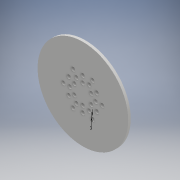
# Autodesk Inventor part: bottom-bearing-holder
Saved by Autodesk Inventor 2018 (Build 220112000, 112)
## iProperties
Created: 2024-05-26
Part Number: bottom-bearing-holder
Material: Generic
Document SubType Name: Modeling
Designer: neo
Density: 1 g/cm^3
Appearance: Default
Author: neo
Autodesk Inventor part; units mm, degrees
ref_plane "YZ Plane" through (0, 0, 0) normal (1, 0, 0) x (0, 1, 0)
ref_plane "XZ Plane" through (0, 0, 0) normal (0, 1, 0) x (-1, 0, 0)
ref_plane "XY Plane" through (0, 0, 0) normal (0, 0, 1) x (1, 0, 0)
sketch "Sketch1" plane through (0, 0, 0) normal (0, 0, 1) x (1, 0, 0)
  line L0 (0, 30.0543) -> (0, -31.5761)
  line L1 (40, 7.4457) -> (50, 7.4457)
  line L2 (50, 7.4457) -> (50, -2.5543)
  line L3 (50, -2.5543) -> (40, -2.5543)
  line L4 (40, -2.5543) -> (40, 7.4457)
  point P0 (0, 0)
  dimension "d0" = 10
  dimension "d1" = 10
  dimension "d2" = 80
  constraints: 10 end point, 2 parallel, 1 horizontal, 1 perpendicular, 1 point on line, 1 vertical
  measures "d0" distance of L1.start L1.end
  measures "d1" distance of L1.end L2.end
  measures "d2" diameter of L4 L0
revolve "Revolution1" add sketch "Sketch1" angle 360 about axis through (0, 30.0543, 0) along (0, -1, 0)
sketch "Sketch3" plane through (0, 7.4457, 0) normal (0, 1, 0) x (1, 0, 0)
  circle A0 centre (0, 0) radius 40 projected
  circle A1 centre (0, 0) radius 43
  point P0 (0, 0)
  dimension "d6" = 3
  constraints: 1 centre point, 1 coincident
  measures "d6" radial gap between concentric circles of A0 A1
extrude "Extrusion1" add sketch "Sketch3" along normal blind 4 contours A0 | A1
extrude "Extrusion2" add sketch "Sketch3" against normal blind 4 contours A0
sketch "Sketch4" plane through (0, -2.5543, 0) normal (0, -1, 0) x (1, 0, 0)
  circle A0 centre (0, 0) radius 40 projected
  circle A1 centre (0, 0) radius 43 projected
  point P0 (0, 0)
extrude "Extrusion3" add sketch "Sketch4" against normal blind 4 contours A0
extrude "Extrusion4" add sketch "Sketch4" along normal blind 4 contours A0 | A1
sketch "Sketch5" plane through (0, -6.5543, 0) normal (0, -1, 0) x (1, 0, 0)
  circle A0 centre (0, 0) radius 70
  dimension "d16" = 140
  constraints: 1 centre point, 1 coincident
  measures "d16" diameter of A0
extrude "Extrusion5" add sketch "Sketch5" along normal blind 4
sketch "Sketch6" plane through (0, 11.4457, 0) normal (0, 1, 0) x (1, 0, 0)
  circle A0 centre (0, 0) radius 30
  circle A1 centre (-30, 0) radius 1.5
  line L0 (0, 0) -> (-60.6002, 0)
  line L1 (0, 0) -> (-52.4813, -30.3001)
  line L2 (0, 0) -> (-30.3001, -52.4813)
  line L3 (0, 0) -> (0, -60.6002)
  line L4 (0, 0) -> (30.3001, -52.4813)
  line L5 (0, 0) -> (52.4813, -30.3001)
  line L6 (0, 0) -> (60.6002, 0)
  line L7 (0, 0) -> (52.4813, 30.3001)
  line L8 (0, 0) -> (30.3001, 52.4813)
  line L9 (0, 0) -> (0, 60.6002)
  line L10 (0, 0) -> (-30.3001, 52.4813)
  line L11 (0, 0) -> (-52.4813, 30.3001)
  circle A2 centre (0, 0) radius 20
  circle A3 centre (0, 0) radius 25
  circle A4 centre (0, 0) radius 15
  circle A5 centre (-21.6506, 12.5) radius 1.5
  circle A6 centre (-20, 0) radius 1.5
  circle A7 centre (-12.9904, 7.5) radius 1.5
  circle A8 centre (-15, -25.9808) radius 1.5
  circle A9 centre (-10, -17.3205) radius 1.5
  circle A10 centre (-21.6506, -12.5) radius 1.5
  circle A11 centre (-12.9904, -7.5) radius 1.5
  circle A12 centre (15, -25.9808) radius 1.5
  circle A13 centre (10, -17.3205) radius 1.5
  circle A14 centre (0, -25) radius 1.5
  circle A15 centre (0, -15) radius 1.5
  circle A16 centre (30, 0) radius 1.5
  circle A17 centre (20, 0) radius 1.5
  circle A18 centre (21.6506, -12.5) radius 1.5
  circle A19 centre (12.9904, -7.5) radius 1.5
  circle A20 centre (15, 25.9808) radius 1.5
  circle A21 centre (10, 17.3205) radius 1.5
  circle A22 centre (21.6506, 12.5) radius 1.5
  circle A23 centre (12.9904, 7.5) radius 1.5
  circle A24 centre (-15, 25.9808) radius 1.5
  circle A25 centre (-10, 17.3205) radius 1.5
  circle A26 centre (0, 25) radius 1.5
  circle A27 centre (0, 15) radius 1.5
  dimension "d19" = 60
  dimension "d25" = 40
  dimension "d26" = 50
  dimension "d27" = 30
  dimension "d20" = 3
  dimension "d23" = 360
  dimension "d28" = 3
  dimension "d29" = 3
  dimension "d30" = 3
  dimension "d33" = 360
  constraints: 24 centre point, 24 end point, 5 point on line, 3 coincident, 2 horizontal alignment, 1 horizontal, 96 other
  measures "d20" diameter of A1
  measures "d28" diameter of A5
  measures "d29" diameter of A6
  measures "d30" diameter of A7
hole "Hole1" at (-15, 11.4457, 25.9808) at (-30, 11.4457, 0) at (-15, 11.4457, -25.9808) at (15, 11.4457, -25.9808) at (30, 11.4457, 0) at (15, 11.4457, 25.9808) at (0, 11.4457, 25) at (-21.6506, 11.4457, 12.5) at (-21.6506, 11.4457, -12.5) at (-10, 11.4457, -17.3205) at (10, 11.4457, -17.3205) at (20, 11.4457, 0) at (21.6506, 11.4457, 12.5) at (21.6506, 11.4457, -12.5) at (12.9904, 11.4457, -7.5) at (12.9904, 11.4457, 7.5) at (10, 11.4457, 17.3205) at (0, 11.4457, 15) at (-10, 11.4457, 17.3205) at (-12.9904, 11.4457, 7.5) at (-20, 11.4457, 0) at (-12.9904, 11.4457, -7.5) at (0, 11.4457, -15) at (0, 11.4457, -25) direction (0, -1, 0) diameter 3 end through all counterbore diameter 6 counterbore depth 4
sketch "Sketch7" plane through (0, -10.5543, 0) normal (0, -1, 0) x (1, 0, 0)
  circle A0 centre (0, -15) radius 1.5 projected
  circle A1 centre (-20, 0) radius 1.5 projected
  circle A2 centre (-10, 17.3205) radius 1.5 projected
  circle A3 centre (10, 17.3205) radius 1.5 projected
  circle A4 centre (12.9904, -7.5) radius 1.5 projected
  circle A5 centre (21.6506, 12.5) radius 1.5 projected
  circle A6 centre (10, -17.3205) radius 1.5 projected
  circle A7 centre (-21.6506, -12.5) radius 1.5 projected
  circle A8 centre (0, 25) radius 1.5 projected
  circle A9 centre (30, 0) radius 1.5 projected
  circle A10 centre (-15, -25.9808) radius 1.5 projected
  circle A11 centre (-15, 25.9808) radius 1.5 projected
  circle A12 centre (-30, 0) radius 1.5 projected
  circle A13 centre (15, -25.9808) radius 1.5 projected
  circle A14 centre (15, 25.9808) radius 1.5 projected
  circle A15 centre (-21.6506, 12.5) radius 1.5 projected
  circle A16 centre (-10, -17.3205) radius 1.5 projected
  circle A17 centre (20, 0) radius 1.5 projected
  circle A18 centre (21.6506, -12.5) radius 1.5 projected
  circle A19 centre (12.9904, 7.5) radius 1.5 projected
  circle A20 centre (0, 15) radius 1.5 projected
  circle A21 centre (-12.9904, 7.5) radius 1.5 projected
  circle A22 centre (-12.9904, -7.5) radius 1.5 projected
  circle A23 centre (0, -25) radius 1.5 projected
  circle A24 centre (0, 0) radius 70 projected
  point P0 (0, 0)
hole "Hole2" at (30, -10.5543, 0) at (21.6506, -10.5543, -12.5) at (20, -10.5543, 0) at (21.6506, -10.5543, 12.5) at (15, -10.5543, 25.9808) at (12.9904, -10.5543, 7.5) at (12.9904, -10.5543, -7.5) at (15, -10.5543, -25.9808) at (10, -10.5543, -17.3205) at (0, -10.5543, -15) at (0, -10.5543, -25) at (0, -10.5543, 15) at (0, -10.5543, 25) at (10, -10.5543, 17.3205) at (-10, -10.5543, 17.3205) at (-15, -10.5543, 25.9808) at (-12.9904, -10.5543, 7.5) at (-21.6506, -10.5543, 12.5) at (-20, -10.5543, 0) at (-30, -10.5543, 0) at (-12.9904, -10.5543, -7.5) at (-21.6506, -10.5543, -12.5) at (-15, -10.5543, -25.9808) at (-10, -10.5543, -17.3205) direction (0, 1, 0) diameter 3 end through all counterbore diameter 6 counterbore depth 4
equation "\"d9\" = t"
equation "\"d12\" = t"
equation "\"d14\" = t"
equation "\"d17\" = t"
equation "\"d38\" = t"
equation "\"d45\" = t"
equation "\"t\" = 4"
body "Solid1"
